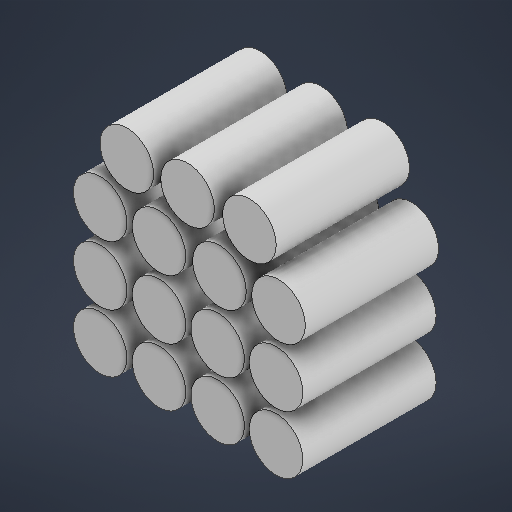
# Autodesk Inventor part: battery_case
Saved by Autodesk Inventor 2026.1 (Build 301233000, 233)
## iProperties
Created: 2025-03-06
Part Number: battery_case
Material: Generic
Document SubType Name: Modeling
Designer: aaron
Density: 1 g/cm^3
Appearance: Default
Author: aaron
Autodesk Inventor part; units mm, degrees
ref_plane "YZ Plane" through (0, 0, 0) normal (1, 0, 0) x (0, 1, 0)
ref_plane "XZ Plane" through (0, 0, 0) normal (0, 1, 0) x (-1, 0, 0)
ref_plane "XY Plane" through (0, 0, 0) normal (0, 0, 1) x (1, 0, 0)
sketch "Sketch1" plane through (0, 0, 0) normal (0, 0, 1) x (1, 0, 0)
  circle A0 centre (-32.3432, 16.2465) radius 13
  circle A1 centre (-3.6418, 16.2465) radius 13
  circle A2 centre (24.9334, 16.2465) radius 13
  circle A3 centre (53.41, 16.2465) radius 13
  circle A4 centre (-32.3432, 44.5158) radius 13
  circle A5 centre (-3.6418, 44.5158) radius 13
  circle A6 centre (24.9334, 44.5158) radius 13
  circle A7 centre (53.41, 44.5158) radius 13
  circle A8 centre (-3.6418, 73.4238) radius 13
  circle A9 centre (10.2637, 100.3902) radius 13
  circle A10 centre (40.41, 100.3902) radius 13
  circle A11 centre (-32.3432, 73.4238) radius 13
  circle A12 centre (25.7964, 73.4238) radius 13
  circle A13 centre (54.5965, 73.4238) radius 13
  circle A14 centre (-19.3432, 100.3902) radius 13
  point P0 (0, 0)
  dimension "d0" = 26
  dimension "d2" = 26
  dimension "d4" = 26
  dimension "d17" = 26
  dimension "d19" = 26
  dimension "d20" = 26
  dimension "d21" = 26
  dimension "d22" = 26
  dimension "d24" = 26
  dimension "d25" = 26
  dimension "d26" = 26
  dimension "d28" = 26
  dimension "d29" = 26
  dimension "d30" = 26
  dimension "d31" = 26
  constraints: 15 centre point
  measures "d0" diameter of A0
  measures "d2" diameter of A1
  measures "d4" diameter of A2
  measures "d17" diameter of A3
  measures "d19" diameter of A4
  measures "d20" diameter of A5
  measures "d21" diameter of A6
  measures "d22" diameter of A7
  measures "d24" diameter of A8
  measures "d25" diameter of A9
  measures "d26" diameter of A10
  measures "d28" diameter of A11
  measures "d29" diameter of A12
  measures "d30" diameter of A13
  measures "d31" diameter of A14
extrude "Extrusion1" add sketch "Sketch1" along normal blind 65
equation "\"d2\" = d0"
equation "\"d4\" = d0"
body "Solid1"
